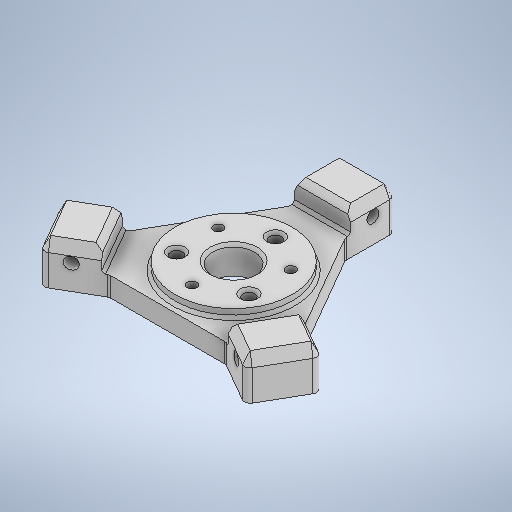
# Autodesk Inventor part: Base_E_buffer
Saved by Autodesk Inventor 2025 (Build 290162000, 162)
## iProperties
Created: 2026-06-13
Part Number: Base_E_buffer
Material: Generic
Document SubType Name: Sheet Metal
Designer: MSI
Density: 1 g/cm^3
Sheet Metal Rule: Default_mm
Appearance: Default
Author: MSI
Autodesk Inventor part; units mm, degrees
ref_plane "YZ Plane" through (0, 0, 0) normal (1, 0, 0) x (0, 1, 0)
ref_plane "XZ Plane" through (0, 0, 0) normal (0, 1, 0) x (-1, 0, 0)
ref_plane "XY Plane" through (0, 0, 0) normal (0, 0, 1) x (1, 0, 0)
sketch "Sketch1" plane through (0, 0, 0) normal (0, 1, 0) x (-1, 0, 0)
  line L0 (0, -40) -> (0, 0)
  line L1 (29.641, 28.6603) -> (21.4449, 23.9282)
  line L2 (39.641, 11.3397) -> (31.4449, 6.6077)
  line L3 (20.4449, 23.6603) -> (-20.4449, 23.6603)
  line L4 (-30.7128, 5.8756) -> (-10.2679, -29.5359)
  line L5 (10.2679, -29.5359) -> (30.7128, 5.8756)
  arc A0 (20.4449, 23.6603) -> (21.4449, 23.9282) centre (20.4449, 25.6603) ccw
  arc A1 (31.4449, 6.6077) -> (30.7128, 5.8756) centre (32.4449, 4.8756) ccw
  arc A2 (10.2679, -29.5359) -> (10, -30.5359) centre (12, -30.5359) ccw
  arc A3 (-30.7128, 5.8756) -> (-31.4449, 6.6077) centre (-32.4449, 4.8756) ccw
  arc A4 (-21.4449, 23.9282) -> (-20.4449, 23.6603) centre (-20.4449, 25.6603) ccw
  arc A5 (-10, -30.5359) -> (-10.2679, -29.5359) centre (-12, -30.5359) ccw
  arc A6 (-28.541, 28.0252) -> (-38.541, 10.7047) centre (0, 0) ccw
  arc A7 (-10, -38.7298) -> (10, -38.7298) centre (0, 0) ccw
  arc A8 (38.541, 10.7047) -> (28.541, 28.0252) centre (0, 0) ccw
  circle A9 centre (0, 0) radius 21
  circle A10 centre (0, 0) radius 7.5
  circle A11 centre (0, -15) radius 2.1
  circle A12 centre (-12.9904, -7.5) radius 1.75
  line L6 (0, -40) -> (0, -32)
  line L7 (0, -32) -> (0, -48)
  line L8 (0, -48) -> (-8, -48)
  line L9 (-10, -46) -> (-10, -32)
  line L10 (-10, -32) -> (10, -32)
  line L11 (10, -32) -> (10, -46)
  line L12 (8, -48) -> (0, -48)
  line L13 (-10, -32) -> (-10, -30.5359)
  line L14 (10, -32) -> (10, -30.5359)
  arc A13 (8, -48) -> (10, -46) centre (8, -46) ccw
  arc A14 (-10, -46) -> (-8, -48) centre (-8, -46) ccw
  arc A15 (31.4449, 6.6077) -> (30.7128, 5.8756) centre (32.4449, 4.8756) ccw
  arc A16 (20.4449, 23.6603) -> (21.4449, 23.9282) centre (20.4449, 25.6603) ccw
  line L15 (22.7128, 24.6603) -> (21.4449, 23.9282)
  line L16 (32.7128, 7.3397) -> (31.4449, 6.6077)
  line L17 (32.7128, 7.3397) -> (22.7128, 24.6603)
  line L18 (34.641, 20) -> (27.7128, 16)
  arc A17 (38.541, 10.7047) -> (28.541, 28.0252) centre (0, 0) ccw
  line L19 (22.7128, 24.6603) -> (34.8372, 31.6603)
  line L20 (44.8372, 14.3397) -> (32.7128, 7.3397)
  line L21 (27.7128, 16) -> (41.5692, 24)
  arc A18 (44.8372, 14.3397) -> (45.5692, 17.0718) centre (43.8372, 16.0718) ccw
  line L22 (41.5692, 24) -> (45.5692, 17.0718)
  line L23 (37.5692, 30.9282) -> (41.5692, 24)
  arc A19 (37.5692, 30.9282) -> (34.8372, 31.6603) centre (35.8372, 29.9282) ccw
  arc A20 (-21.4449, 23.9282) -> (-20.4449, 23.6603) centre (-20.4449, 25.6603) ccw
  arc A21 (-30.7128, 5.8756) -> (-31.4449, 6.6077) centre (-32.4449, 4.8756) ccw
  line L24 (-32.7128, 7.3397) -> (-31.4449, 6.6077)
  line L25 (-22.7128, 24.6603) -> (-21.4449, 23.9282)
  line L26 (-22.7128, 24.6603) -> (-32.7128, 7.3397)
  line L27 (-34.641, 20) -> (-27.7128, 16)
  arc A22 (-28.541, 28.0252) -> (-38.541, 10.7047) centre (0, 0) ccw
  line L28 (-32.7128, 7.3397) -> (-44.8372, 14.3397)
  line L29 (-34.8372, 31.6603) -> (-22.7128, 24.6603)
  line L30 (-27.7128, 16) -> (-41.5692, 24)
  arc A23 (-34.8372, 31.6603) -> (-37.5692, 30.9282) centre (-35.8372, 29.9282) ccw
  line L31 (-41.5692, 24) -> (-37.5692, 30.9282)
  line L32 (-45.5692, 17.0718) -> (-41.5692, 24)
  arc A24 (-45.5692, 17.0718) -> (-44.8372, 14.3397) centre (-43.8372, 16.0718) ccw
  circle A25 centre (12.9904, 7.5) radius 2.1
  circle A26 centre (-12.9904, 7.5) radius 2.1
  circle A27 centre (12.9904, -7.5) radius 1.75
  circle A28 centre (0, 15) radius 1.75
  point P0 (-10, -45)
  point P1 (30.9808, 6.3397)
  point P2 (10, -48)
  point P3 (43.9711, 13.8397)
  point P4 (36.5692, 32.6603)
  point P5 (-33.9711, 31.1603)
  point P6 (-46.5692, 15.3397)
  dimension "d22" = 2
  dimension "d23" = 42
  dimension "d74" = 2
  dimension "d77" = 360
  dimension "d81" = 360
  dimension "d86" = 360
  dimension "d88" = 15
  constraints: 66 end point, 42 point on circle, 29 centre point, 16 point on line, 12 tangent, 6 equal radius, 5 coincident, 5 perpendicular, 1 horizontal, 1 parallel, 1 vertical, 124 other
  measures "d22" radius of A0
  measures "d23" diameter of A9
  measures "d74" radius of A13
  measures "d88" diameter of A10
extrude "Extrusion5" add sketch "Sketch1" along normal blind 7 contours L10 L13 A5 L4 A3 L24 L26 L25 A4 L3 A0 L1 L17 L2 A1 L5 A2 L14
extrude "Extrusion6" add sketch "Sketch1" along normal blind 10 contours A9
extrude "Extrusion7" add sketch "Sketch1" along normal blind 15 contours A7 L9 L10 L0 | L7 L8 A14 L9 A7 | L0 L10 L11 A7 | A7 L11 A13 L12 L7 | L28 A6 L27 L26 | L17 L18 A8 L2 | L27 A6 L29 L26 | L28 A24 L32 L30 A6 | A8 L21 L22 A18 L20 L2 | L17 L1 A8 L18 | L30 L31 A23 L29 A6 | A8 L1 L19 A19 L23 L21
chamfer "Chamfer6" distance 2 distance2 4 5 edges at (-28.775, 15, 28.1603) (-36.3548, 15, 31.8601) (-41.5692, 15, 24) (-45.769, 15, 15.5542) (-38.775, 15, 10.8397) measured on face at (-38.525, 15, 11.2728) measured on face at (-36.2254, 15, 31.3771) measured on face at (-45.2861, 15, 15.6836) measured on face at (-41.1362, 15, 23.75) measured on face at (-29.025, 15, 27.7272)
chamfer "Chamfer7" distance 2 distance2 4 5 edges at (28.775, 15, 28.1603) (36.3548, 15, 31.8601) (41.5692, 15, 24) (45.769, 15, 15.5542) (38.775, 15, 10.8397) measured on face at (29.025, 15, 27.7272) measured on face at (41.1362, 15, 23.75) measured on face at (38.525, 15, 11.2728) measured on face at (36.2254, 15, 31.3771) measured on face at (45.2861, 15, 15.6836)
chamfer "Chamfer8" distance 2 distance2 4 5 edges at (10, 15, -39) (9.4142, 15, -47.4142) (0, 15, -48) (-9.4142, 15, -47.4142) (-10, 15, -39) measured on face at (0, 15, -47.5) measured on face at (-9.0607, 15, -47.0607) measured on face at (9.5, 15, -39) measured on face at (9.0607, 15, -47.0607) measured on face at (-9.5, 15, -39)
sketch "Sketch4" plane through (21.4449, 0, 23.9282) normal (-0.5, 0, 0.8660254) x (0.8660254, 0, 0.5)
  circle A0 centre (9.4641, 8.8) radius 2.15
  line L0 (17.4641, 0) -> (17.4641, 11) projected
  line L1 (15.4641, 15) -> (1.4641, 15) projected
  point P0 (-30.5359, 0)
  dimension "d105" = 8
  dimension "d106" = 6.2
  constraints: 1 centre point
  measures "d105" distance from line of L0 A0.centre
  measures "d106" distance from line of L1 A0.centre
extrude "Extrusion8" cut sketch "Sketch4" against normal blind 30
pattern_circular "Circular Pattern2" count 3 over 360 about axis through (0, 0, 0) along (0, 1, 0) of "Extrusion8"
chamfer "Chamfer9" distance 1 angle 45 8 edges at (-27.7128, 7, 16) (0, 7, -32) (27.7128, 7, 16) (21, 7, 0) (7.5, 10, 0) (2.1, 10, -15) (-10.8904, 10, 7.5) (15.0904, 10, 7.5)
chamfer "Chamfer10" distance 2 angle 45 3 edges at (0, 15, -32) (-27.7128, 15, 16) (27.7128, 15, 16)
sketch "Sketch5" plane through (10, 0, -30.5359) normal (1, 0, 0) x (0, 0, -1)
  point P0 (-30.5359, 0)
equation "\"BendRadius\" = Thickness"
equation "\"BendReliefWidth\" = Thickness"
equation "\"BendReliefDepth\" = 0.5 * Thickness"
equation "\"CornerReliefSize\" = 4 * Thickness"
equation "\"MinimumRemnant\" = 2 * Thickness"
equation "\"TransitionRadius\" = BendRadius"
equation "\"JacobiRadiusSize\" = BendRadius"
equation "\"GapSize\" = Thickness"
equation "\"Thickness\" = 0.5"
body "Solid2"
